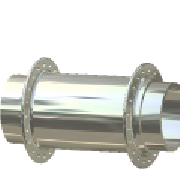
# Autodesk Inventor part: RearHub
Saved by Autodesk Inventor 2012 (Build 160160000, 160)
## iProperties
Created: 2001-05-25
Part Number: RearHub
Document SubType Name: Modeling
Designer: Administrator
Material: Default
Density: 1 g/cm^3
Control State: 0
Master: False
Checked Out: False
Shininess: 86.0
Length Units: 11272
Angle Units: 11279
Time Units: 11290
Mass Units: 11286
Length Display Precision: 3
Angle Display Precision: 2
Compacted: True
Density: 0.0
Volumn: 0.0
Area: 0.0
PropertySet Name: Model Information
Author: Administrator
Autodesk Inventor part; units mm, degrees
ref_plane "YZ Plane" through (0, 0, 0) normal (1, 0, 0) x (0, 1, 0)
ref_plane "XZ Plane" through (0, 0, 0) normal (0, 1, 0) x (-1, 0, 0)
ref_plane "XY Plane" through (0, 0, 0) normal (0, 0, 1) x (1, 0, 0)
sketch "Sketch1" plane through (0, 0, 0) normal (0, 0, 1) x (1, 0, 0)
  line L0 (0, -4.874) -> (0, 63.3624) projected
  line L1 (-95.25, 0) -> (127, 0) projected
  line L2 (0, 23.8125) -> (53.975, 23.8125)
  line L3 (53.975, 23.8125) -> (53.975, 28.067)
  line L4 (53.975, 28.067) -> (79.375, 28.067)
  line L5 (79.375, 28.067) -> (79.375, 31.75)
  line L6 (79.375, 31.75) -> (60.325, 31.75)
  line L7 (60.325, 31.75) -> (60.325, 34.925)
  line L8 (60.325, 34.925) -> (56.2687, 34.925)
  arc A0 (52.5503, 38.6434) -> (56.2687, 34.925) centre (56.2687, 38.6434) ccw
  line L9 (52.5503, 38.6434) -> (52.5503, 46.99)
  arc A1 (52.5503, 46.99) -> (49.0497, 46.99) centre (50.8, 46.99) ccw
  line L10 (49.0497, 46.99) -> (49.0497, 38.6434)
  arc A2 (45.3313, 34.925) -> (49.0497, 38.6434) centre (45.3313, 38.6434) ccw
  line L11 (45.3313, 34.925) -> (0, 34.925)
  line L12 (0, 34.925) -> (0, 23.8125)
  line L13 (0, 23.8125) -> (-53.975, 23.8125)
  line L14 (-53.975, 23.8125) -> (-53.975, 28.067)
  line L15 (-53.975, 28.067) -> (-79.375, 28.067)
  line L16 (-79.375, 28.067) -> (-79.375, 31.75)
  line L17 (-79.375, 31.75) -> (-60.325, 31.75)
  line L18 (-60.325, 31.75) -> (-60.325, 34.925)
  line L19 (-60.325, 34.925) -> (-56.2687, 34.925)
  arc A3 (-56.2687, 34.925) -> (-52.5503, 38.6434) centre (-56.2687, 38.6434) ccw
  line L20 (-52.5503, 38.6434) -> (-52.5503, 46.99)
  arc A4 (-49.0497, 46.99) -> (-52.5503, 46.99) centre (-50.8, 46.99) ccw
  line L21 (-49.0497, 46.99) -> (-49.0497, 38.6434)
  arc A5 (-49.0497, 38.6434) -> (-45.3313, 34.925) centre (-45.3313, 38.6434) ccw
  line L22 (-45.3313, 34.925) -> (0, 34.925)
  line L23 (0, 34.925) -> (0, 23.8125)
  point P0 (0, 0)
  dimension "d0" = 158.75
  dimension "d1" = 3.5007
  dimension "d2" = 3.7184
  dimension "d3" = 101.6
  dimension "d4" = 63.5
  dimension "d5" = 12.065
  dimension "d6" = 3.175
  dimension "d17" = 120.65
  dimension "d18" = 107.95
  dimension "d19" = 56.134
  dimension "d20" = 47.625
  constraints: 44 end point, 15 symmetric about line, 12 point on circle, 6 centre point, 6 tangent, 4 vertical, 3 horizontal, 2 collinear, 2 point on line, 1 equal radius, 14 other
  measures "d0" diameter of L5 L0
  measures "d1" diameter of A1
  measures "d2" radius of A2
  measures "d3" diameter of A1.centre L0
  measures "d4" diameter of L6 L1
  measures "d5" distance from line of A1.centre L11
  measures "d6" distance of L6.end L7.end
  measures "d17" distance between parallel lines of L7 L18
  measures "d18" diameter of L3 L0
  measures "d19" diameter of L15 L1
  measures "d20" diameter of L13 L1
revolve "Revolution1" add sketch "Sketch1" angle 360 about axis through (-10, 0, 0) along (1, 0, 0)
sketch "Sketch2" plane through (0, 0, 0) normal (1, 0, 0) x (0, 1, 0)
  line L0 (-4.4055, 0) -> (57.2709, 0) projected
  line L1 (0, -9.6696) -> (0, 5.2233) projected
  line L2 (0, 0) -> (41.8909, 0)
  line L3 (0, 0) -> (41.5052, -6.5738)
  arc A0 (41.5052, -6.5738) -> (42.0226, 0) centre (0, 0) ccw
  circle A1 centre (42.0226, 0) radius 2.032
  circle A2 centre (41.5052, -6.5738) radius 2.032
  dimension "d8" = 9
  dimension "d9" = 4.064
  constraints: 4 end point, 3 centre point, 3 coincident, 2 point on circle, 2 point on line, 1 equal radius
  measures "d8" angle of L3 L2
  measures "d9" diameter of A2
extrude "Extrusion1" cut sketch "Sketch2" along normal through all contours L0 A1 | L0 A0 A1 | L0 A1 A0
extrude "Extrusion2" cut sketch "Sketch2" against normal through all contours A2 L3 A0 | A0 L3 A2
pattern_circular "Circular Pattern1" count 20 over 360 about axis through (22.6656, 0, 0) along (1, 0, 0) of "Extrusion2", "Extrusion1"
body "Solid1"
